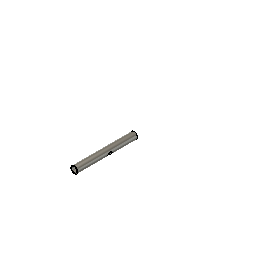
Axis3tube (Autodesk Fusion 360 design; units mm, degrees)
Autodesk Fusion 360 part; units mm, degrees
sketch "Sketch1" plane through (0, 0, 0) normal (0, 0, 1) x (1, 0, 0)
  circle A0 centre (80, -10) radius 4
  circle A1 centre (80, -10) radius 3
  arc A2 (75.981, -10.5) -> (84.019, -10.5) centre (80, -10) ccw
  dimension "d621" = 1
  dimension "d622" = 8
  measures "d621" distance of A0 A1
  measures "d622" diameter of A0
extrude "Extrude1" add sketch "Sketch1" along normal up to surface (39 mm away) and the other way up to surface (31 mm away)
sketch "Sketch2" plane through (71, 0, 0) normal (-1, 0, 0) x (0, 0, 1)
  circle A0 centre (19, 10) radius 3
  line L0 (11.5, -35) -> (11.5, -27)
  arc A1 (11.5, -35) -> (11.5, -27) centre (11.5, -31) ccw
  arc A2 (-17.5, -27) -> (-17.5, -35) centre (-17.5, -31) ccw
  line L1 (-17.5, -27) -> (-17.5, -35)
  line L2 (11.5, 15.5) -> (7.5131, 15.5)
  arc A3 (-13.5131, 15.5) -> (7.5131, 15.5) centre (-3, 16) ccw
  line L3 (-13.5131, 15.5) -> (-17.5, 15.5)
  arc A4 (-17.5, 16.5) -> (-17.5, 15.5) centre (-17.5, 16) ccw
  line L4 (-17.5, 16.5) -> (-13.5131, 16.5)
  arc A5 (7.5131, 16.5) -> (-13.5131, 16.5) centre (-3, 16) ccw
  line L5 (7.5131, 16.5) -> (11.5, 16.5)
  arc A6 (11.5, 15.5) -> (11.5, 16.5) centre (11.5, 16) ccw
  circle A7 centre (19, -10) radius 1.25
  line L6 (-14.25, -32.5) -> (-14.25, -29.5)
  arc A8 (8.25, -29.5) -> (-14.25, -29.5) centre (-3, -29.5) ccw
  line L7 (8.25, -29.5) -> (8.25, -32.5)
  arc A9 (-14.25, -32.5) -> (8.25, -32.5) centre (-3, -32.5) ccw
  line L8 (7, -44) -> (7, -41)
  arc A10 (10, -41) -> (7, -41) centre (8.5, -41) ccw
  line L9 (10, -41) -> (10, -44)
  arc A11 (7, -44) -> (10, -44) centre (8.5, -44) ccw
  line L10 (7, -21) -> (7, -18)
  arc A12 (10, -18) -> (7, -18) centre (8.5, -18) ccw
  line L11 (10, -18) -> (10, -21)
  arc A13 (7, -21) -> (10, -21) centre (8.5, -21) ccw
  line L12 (-16, -44) -> (-16, -41)
  arc A14 (-13, -41) -> (-16, -41) centre (-14.5, -41) ccw
  line L13 (-13, -41) -> (-13, -44)
  arc A15 (-16, -44) -> (-13, -44) centre (-14.5, -44) ccw
  line L14 (-16, -21) -> (-16, -18)
  arc A16 (-13, -18) -> (-16, -18) centre (-14.5, -18) ccw
  line L15 (-13, -18) -> (-13, -21)
  arc A17 (-16, -21) -> (-13, -21) centre (-14.5, -21) ccw
  spline S0 degree 3 poles (-25, 20.4738) (-25, 20.578) (-24.9763, 20.7009) (-24.899, 20.8921) (-24.8324, 20.9949) (-24.6917, 21.139) (-24.5934, 21.2067) (-24.412, 21.2836) (-24.2975, 21.307) (-24.2, 21.307) knots 0.363121 0.363121 0.363121 0.363121 0.394402 0.394402 0.425005 0.425005 0.454845 0.454845 0.484084 0.484084 0.484084 0.484084
  line L16 (-25, 20.4738) -> (-25, -40.4738)
  spline S1 degree 3 poles (-24.2, -41.307) (-24.2975, -41.307) (-24.412, -41.2836) (-24.5934, -41.2067) (-24.6917, -41.139) (-24.8324, -40.9949) (-24.899, -40.8921) (-24.9763, -40.7009) (-25, -40.578) (-25, -40.4738) knots 0.484084 0.484084 0.484084 0.484084 0.513322 0.513322 0.543163 0.543163 0.573765 0.573765 0.605046 0.605046 0.605046 0.605046
  line L17 (-24.2, -41.307) -> (-22, -41.307)
  line L18 (-22, -41.307) -> (-22, -49.4018)
  spline S2 degree 3 poles (-21.9486, -49.9687) (-21.9838, -49.7763) (-22, -49.5812) (-22, -49.4018) knots 0.395834 0.395834 0.395834 0.395834 0.449674 0.449674 0.449674 0.449674
  line L19 (-21.9486, -49.9687) -> (15.9486, -49.9687)
  spline S3 degree 3 poles (16, -49.4018) (16, -49.5812) (15.9838, -49.7763) (15.9486, -49.9687) knots 1.350544 1.350544 1.350544 1.350544 1.404371 1.404371 1.404371 1.404371
  line L20 (16, -49.4018) -> (16, -41.307)
  line L21 (16, -41.307) -> (23.2, -41.307)
  spline S4 degree 3 poles (24, -40.4738) (24, -40.578) (23.9763, -40.7009) (23.899, -40.8921) (23.8324, -40.9949) (23.6917, -41.139) (23.5934, -41.2067) (23.412, -41.2836) (23.2975, -41.307) (23.2, -41.307) knots 0.363121 0.363121 0.363121 0.363121 0.394402 0.394402 0.425005 0.425005 0.454845 0.454845 0.484084 0.484084 0.484084 0.484084
  line L22 (24, -40.4738) -> (24, 20.4738)
  spline S5 degree 3 poles (23.2, 21.307) (23.2975, 21.307) (23.412, 21.2836) (23.5934, 21.2067) (23.6917, 21.139) (23.8324, 20.9949) (23.899, 20.8921) (23.9763, 20.7009) (24, 20.578) (24, 20.4738) knots 0.484084 0.484084 0.484084 0.484084 0.513322 0.513322 0.543163 0.543163 0.573765 0.573765 0.605046 0.605046 0.605046 0.605046
  line L23 (23.2, 21.307) -> (16, 21.307)
  line L24 (16, 21.307) -> (16, 29.4018)
  spline S6 degree 3 poles (15.9486, 29.9687) (15.9838, 29.7763) (16, 29.5812) (16, 29.4018) knots 0.395848 0.395848 0.395848 0.395848 0.449675 0.449675 0.449675 0.449675
  line L25 (15.9486, 29.9687) -> (-21.9486, 29.9687)
  spline S7 degree 3 poles (-22, 29.4018) (-22, 29.5812) (-21.9838, 29.7763) (-21.9486, 29.9687) knots 1.350544 1.350544 1.350544 1.350544 1.404384 1.404384 1.404384 1.404384
  line L26 (-22, 29.4018) -> (-22, 21.307)
  line L27 (-22, 21.307) -> (-24.2, 21.307)
  circle A18 centre (19, -10) radius 1.25
extrude "Extrude2" cut sketch "Sketch2" along normal up to surface contours A7 A18 end surface at (78.6314, -12.6696, 26)
sketch "Sketch3" plane through (80, -10, -29) normal (-0.866025, 0.5, 0) x (0, 0, 1)
  circle A0 centre (30, 0) radius 3
  arc A1 (26.4432, -1.8301) -> (33.5568, -1.8301) centre (30, 0) ccw
  dimension "d631" = 6
  measures "d631" diameter of A0
extrude "Extrude3" cut sketch "Sketch3" against normal blind 7
chamfer "Chamfer1" distance 0.5 angle 45 1 edges at (77.203, -8.9152, -31)
